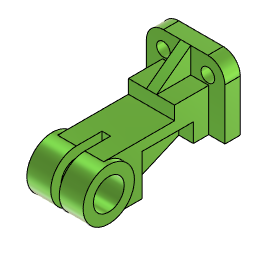
Exercise-12 v0 (Autodesk Fusion 360 design; units mm, degrees)
Autodesk Fusion 360 part; units mm, degrees
sketch "Sketch1" plane through (0, 0, 0) normal (1, 0, 0) x (0, 1, 0)
  circle A0 centre (0, 0) radius 18
  circle A1 centre (0, 0) radius 30
  line L0 (0, 30) -> (83, 30)
  line L1 (83, 30) -> (83, 46)
  line L2 (83, 46) -> (123, 46)
  line L3 (123, 46) -> (123, -4)
  line L4 (123, -4) -> (105, -4)
  line L5 (105, -4) -> (105, 18)
  line L6 (105, 18) -> (45, 18)
  line L7 (45, 18) -> (45, -30)
  line L8 (45, -30) -> (0, -30)
  line L9 (123, -4) -> (141, -4)
  line L10 (141, -4) -> (141, 76)
  line L11 (141, 76) -> (123, 76)
  line L12 (123, 76) -> (123, -4)
  line L13 (83, 46) -> (123, 76)
  line L14 (45, -30) -> (105, -4)
  dimension "d1" = 36
  dimension "d2" = 60
  dimension "d3" = 83
  dimension "d4" = 40
  dimension "d5" = 48
  dimension "d6" = 45
  dimension "d7" = 60
  dimension "d8" = 18
  dimension "d9" = 80
  dimension "d10" = 22
  dimension "d11" = 16
  constraint coincident A0.centre A1.centre
  constraint coincident A1 L0.start
  constraint tangent A1 L0
  constraint horizontal L0
  constraint perpendicular L0 L1
  constraint perpendicular L1 L2
  constraint perpendicular L0 L3
  constraint perpendicular L3 L4
  constraint perpendicular L0 L5
  constraint perpendicular L3 L6
  constraint perpendicular L6 L7
  constraint coincident A1 L8.end
  constraint tangent A1 L8
  constraint perpendicular L7 L8
  constraint horizontal L9
  constraint vertical L10
  constraint horizontal L11
  constraint vertical L12
  measures "d1" diameter of A0
  measures "d2" diameter of A1
  measures "d3" distance of L0.start L0.end
  measures "d4" distance of L1.end L2.end
  measures "d5" distance of L6.end L7.end
  measures "d6" distance of L7.end L8.end
  measures "d7" distance of L5.end L6.end
  measures "d8" distance of L3.end L9.end
  measures "d9" distance of L9.end L10.end
  measures "d10" distance of L4.end L5.end
  measures "d11" distance of L0.end L1.end
extrude "Extrude1" add sketch "Sketch1" along normal mid plane 66 contours A1
extrude "Extrude2" add sketch "Sketch1" along normal mid plane 54 contours A1 L0 L1 L2 L3 L4 L5 L6 L7 L8 L12
extrude "Extrude3" add sketch "Sketch1" along normal mid plane 12 contours L2 L12 L13
extrude "Extrude4" add sketch "Sketch1" along normal mid plane 92 contours L3 L9 L10 L11 L12
extrude "Extrude5" add sketch "Sketch1" along normal mid plane 20 contours L5 L6 L7 L14
fillet "Fillet1" radius 20 2 edges at (46, 132, 76) (-46, 132, 76)
sketch "Sketch2" plane through (0, 0, 30) normal (0, 0, 1) x (-1, 0, 0)
  line L0 (27, 0) -> (-27, 0)
  line L1 (-27, 0) -> (-27, -83)
  line L2 (-27, -83) -> (27, -83)
  line L3 (27, -83) -> (27, 0)
  line L4 (-5, -30) -> (5, -30)
  line L5 (5, -30) -> (5, 30)
  line L6 (5, 30) -> (-5, 30)
  line L7 (-5, 30) -> (-5, -30)
  line L8 (-5, -30) -> (5, 30) construction
  line L9 (5, -30) -> (-5, 30) construction
  dimension "d24" = 10
  dimension "d25" = 60
  constraint horizontal L4
  constraint perpendicular L4 L5
  constraint parallel L4 L6
  constraint parallel L5 L7
  constraint coincident L8 origin
  constraint coincident L9 origin
  measures "d24" distance of L5.end L6.end
  measures "d25" distance of L4 L6
extrude "Extrude6" cut sketch "Sketch2" against normal blind 100 contours L0 L4 L5 L7 | L0 L5 L6 L7
hole "Hole1" at (26, 123, 56) direction (0, 1, 0) diameter 16 end through all
mirror "Mirror1" about plane through (0, 0, 0) normal (1, 0, 0) of "Hole1"
